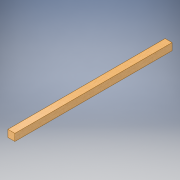
# Autodesk Inventor part: Балясина-01
Saved by Autodesk Inventor 2019 (Build 230136000, 136)
## iProperties
Created: 2018-10-11
Part Number: Балясина-01
Material: Сосна, обыкновенная
Document SubType Name: Modeling
Designer: Андреев Н.Л.
Density: 0.496 g/cm^3
Appearance: Желтая сосна — темное морение — с умеренным глянцем
ШИРИНА: 40
ТОЛЩВЫС: 40
ДЛИНА: 900
Author: Андреев Н.Л.
Autodesk Inventor part; units mm, degrees
ref_plane "YZ Plane" through (0, 0, 0) normal (1, 0, 0) x (0, 1, 0)
ref_plane "XZ Plane" through (0, 0, 0) normal (0, 1, 0) x (-1, 0, 0)
ref_plane "XY Plane" through (0, 0, 0) normal (0, 0, 1) x (1, 0, 0)
sketch "Эскиз1" plane through (0, 0, 0) normal (0, 0, 1) x (1, 0, 0)
  line L0 (-20, -20) -> (20, -20)
  line L1 (20, -20) -> (20, 20)
  line L2 (20, 20) -> (-20, 20)
  line L3 (-20, 20) -> (-20, -20)
  line L4 (-20, -20) -> (20, 20) construction
  line L5 (20, -20) -> (-20, 20) construction
  point P0 (0, 0)
  dimension "ШИРИНА" = 40
  dimension "ТОЛЩВЫС" = 40
  constraints: 12 end point, 2 midpoint, 2 parallel, 1 horizontal, 1 perpendicular
  measures "ШИРИНА" distance of L2.end L1.end
  measures "ТОЛЩВЫС" distance of L1.end L0.end
extrude "Выдавливание1" add sketch "Эскиз1" along normal blind 900
